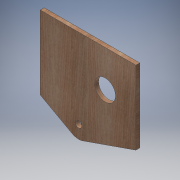
# Autodesk Inventor part: cannonSideWall
Saved by Autodesk Inventor 2018 (Build 220112000, 112)
## iProperties
Created: 2017-05-03
Part Number: cannonSideWall
Material: Generic
Document SubType Name: Modeling
Designer: gsegs
Density: 1 g/cm^3
Appearance: Birch - Natural Polished
Author: gsegs
Autodesk Inventor part; units mm, degrees
ref_plane "YZ Plane" through (0, 0, 0) normal (1, 0, 0) x (0, 1, 0)
ref_plane "XZ Plane" through (0, 0, 0) normal (0, 1, 0) x (-1, 0, 0)
ref_plane "XY Plane" through (0, 0, 0) normal (0, 0, 1) x (1, 0, 0)
ref_plane "Work Plane1" through (-4668.2945, 0, 0) normal (0, 0, 1) x (1, 0, 0)
sketch "Sketch1" plane through (-4668.2945, 0, 0) normal (0, 0, 1) x (1, 0, 0)
  line L0 (0, 19.05) -> (466.725, 19.05) projected
  line L1 (466.725, 0) -> (466.725, 19.05) projected
  line L2 (0, 0) -> (0, 19.05) projected
  line L3 (0, -340.481) -> (0, -321.431) projected
  line L4 (466.725, -340.481) -> (0, -340.481) projected
  line L5 (466.725, -340.481) -> (0, -340.481) projected
  line L6 (466.725, -340.481) -> (466.725, -321.431) projected
  line L7 (0, -321.431) -> (466.725, -321.431) construction
  line L8 (0, -340.481) -> (0, -321.431) projected
  line L9 (466.725, 19.05) -> (0, 19.05)
  line L10 (0, 19.05) -> (0, -340.481)
  line L11 (466.725, -340.481) -> (466.725, 19.05)
  line L12 (147.3639, -408.7465) -> (46.3111, -408.7465) construction
  line L13 (466.725, -340.481) -> (466.725, -408.7465)
  line L14 (466.725, -408.7465) -> (147.3639, -408.7465) construction
  line L15 (46.3111, -408.7465) -> (0, -408.7465)
  line L16 (0, -408.7465) -> (0, -340.481)
  line L17 (466.725, -408.7465) -> (466.725, -434.1465)
  line L18 (466.725, -434.1465) -> (0, -434.1465)
  line L19 (0, -434.1465) -> (0, -408.7465)
  point P0 (4668.2945, 0)
  dimension "d7" = 25.4
  constraints: 22 end point, 5 perpendicular, 3 horizontal, 2 vertical, 1 parallel, 2 other
  measures "d7" distance of L13.end L17.end
extrude "Extrusion1" add sketch "Sketch1" along normal blind 19.05
sketch "Sketch2" plane through (-4668.2945, 0, 0) normal (0, 0, -1) x (-1, 0, 0)
  line L0 (-232.5687, -355.978) -> (-232.5688, 34.547)
  line L1 (-141.2875, -408.7465) -> (-141.2875, 124.6535)
  circle A0 centre (-186.9249, -370.6465) radius 15.875
  line L2 (-232.5687, -370.6465) -> (-141.2875, -370.6465) construction
  line L3 (0, -408.7465) -> (-466.725, -408.7465) projected
  point P0 (-4668.2945, 0)
  dimension "d2" = 31.75
  dimension "d3" = 45.6438
  dimension "d4" = 38.1
  constraints: 6 end point, 3 point on line, 2 vertical, 1 centre point, 1 perpendicular, 4 other
  measures "d2" diameter of A0
  measures "d3" distance from line of L0 A0.centre
  measures "d4" distance between parallel lines of L3 L2
extrude "Extrusion2" cut sketch "Sketch2" against normal up to next
sketch "Sketch3" plane through (-4668.2945, 0, 0) normal (0, 0, -1) x (-1, 0, 0)
  circle A0 centre (-186.9249, -370.6465) radius 15.875 projected
  arc A1 (-207.9625, -430.5603) -> (-155.5881, -425.8756) centre (-186.9249, -370.6465) ccw
  line L0 (0, -434.1465) -> (-466.725, -434.1465) projected
  line L1 (0, -340.481) -> (-157.1625, -426.7397)
  line L2 (-466.725, -340.481) -> (-207.9625, -430.5603)
  line L3 (-466.725, -434.1465) -> (-466.725, -340.481)
  line L4 (-466.725, -434.1465) -> (-466.725, 19.05) projected
  line L5 (0, -434.1465) -> (-466.725, -434.1465) projected
  line L6 (0, -434.1465) -> (0, -340.481)
  line L7 (0, 19.05) -> (0, -434.1465) projected
  arc A2 (-155.5881, -425.8756) -> (-207.9625, -430.5603) centre (-186.9249, -370.6465) ccw construction
  point P0 (-4668.2945, 0)
  point P1 (-186.9249, -434.1465)
  constraints: 8 end point, 6 point on circle, 2 centre point, 2 point on line, 1 collinear, 1 vertical, 3 other
extrude "Extrusion3" cut sketch "Sketch3" against normal blind 19.05 contours A1 L1 L6 L0 | L0 L3 L2 A1
sketch "Sketch4" plane through (-4668.2945, 0, 19.05) normal (0, 0, 1) x (1, 0, 0)
  circle A0 centre (316.7063, -160.7155) radius 12.7 construction
  circle A1 centre (316.7063, -160.7155) radius 50.8
  point P0 (4668.2945, 0)
  dimension "d10" = 101.6
  constraints: 1 centre point, 1 coincident
  measures "d10" diameter of A1
extrude "Extrusion4" cut sketch "Sketch4" against normal up to next
body "Solid1"
